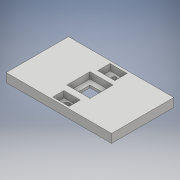
# Autodesk Inventor part: Parte8
Saved by Autodesk Inventor 2017 (Build 210142000, 142)
## iProperties
Part Number: Parte8
Material: Generico
Document SubType Name: Modeling
Designer: Federico
Density: 1 g/cm^3
Appearance: Default
Author: Federico
Autodesk Inventor part; units mm, degrees
ref_plane "YZ Plane" through (0, 0, 0) normal (1, 0, 0) x (0, 1, 0)
ref_plane "XZ Plane" through (0, 0, 0) normal (0, 1, 0) x (-1, 0, 0)
ref_plane "XY Plane" through (0, 0, 0) normal (0, 0, 1) x (1, 0, 0)
sketch "Schizzo1" plane through (0, 0, 0) normal (0, 0, 1) x (1, 0, 0)
  line L0 (-55, 32.5) -> (55, 32.5)
  line L1 (55, 32.5) -> (55, -32.5)
  line L2 (55, -32.5) -> (-55, -32.5)
  line L3 (-55, -32.5) -> (-55, 32.5)
  line L4 (-55, 32.5) -> (55, -32.5) construction
  line L5 (55, 32.5) -> (-55, -32.5) construction
  line L6 (-8.5, -18.7) -> (8.5, -18.7)
  line L7 (8.5, -18.7) -> (8.5, -30.3)
  line L8 (8.5, -30.3) -> (-8.5, -30.3)
  line L9 (-8.5, -30.3) -> (-8.5, -18.7)
  line L10 (-8.5, -18.7) -> (8.5, -30.3) construction
  line L11 (8.5, -18.7) -> (-8.5, -30.3) construction
  line L12 (-12, 12) -> (12, 12)
  line L13 (12, 12) -> (12, -12)
  line L14 (12, -12) -> (-12, -12)
  line L15 (-12, -12) -> (-12, 12)
  line L16 (-12, 12) -> (12, -12) construction
  line L17 (12, 12) -> (-12, -12) construction
  line L18 (-8.95, 29.85) -> (8.95, 29.85)
  line L19 (8.95, 29.85) -> (8.95, 17)
  line L20 (8.95, 17) -> (-8.95, 17)
  line L21 (-8.95, 17) -> (-8.95, 29.85)
  line L22 (-8.95, 29.85) -> (8.95, 17) construction
  line L23 (8.95, 29.85) -> (-8.95, 17) construction
  line L24 (0, 25.425) -> (0, 21.425) construction
  line L25 (-2, 25.425) -> (-2, 21.425)
  line L26 (2, 21.425) -> (2, 25.425)
  arc A0 (2, 25.425) -> (-2, 25.425) centre (0, 25.425) ccw
  arc A1 (-2, 21.425) -> (2, 21.425) centre (0, 21.425) ccw
  circle A2 centre (0, -24.5) radius 4.1
  circle A3 centre (0, 0) radius 3.8
  line L27 (-4, 4) -> (4, 4)
  line L28 (4, 4) -> (4, -4)
  line L29 (4, -4) -> (-4, -4)
  line L30 (-4, -4) -> (-4, 4)
  line L31 (-4, 4) -> (4, -4) construction
  line L32 (4, 4) -> (-4, -4) construction
  point P0 (0, 23.425)
  dimension "d0" = 110
  dimension "d1" = 65
  dimension "d5" = 17
  dimension "d6" = 11.6
  dimension "d8" = 24
  dimension "d9" = 24
  dimension "d11" = 17.9
  dimension "d12" = 12.85
  dimension "d13" = 2
  dimension "d14" = 4
  dimension "d15" = 8.2
  dimension "d16" = 7.6
  dimension "d17" = 8
  dimension "d18" = 8
  constraints: 68 end point, 11 parallel, 10 midpoint, 5 horizontal, 5 perpendicular, 4 centre point, 4 point on circle, 4 tangent, 1 coincident, 1 vertical
  measures "d0" distance of L1.end L2.end
  measures "d1" distance of L0.end L1.end
  measures "d5" distance of L7.end L8.end
  measures "d6" distance of L6.end L7.end
  measures "d8" distance of L13.end L14.end
  measures "d9" distance of L12.end L13.end
  measures "d11" distance of L19.end L20.end
  measures "d12" distance of L18.end L19.end
  measures "d13" distance of point (0, 23.425) L24.end
  measures "d14" diameter of A1
  measures "d15" diameter of A2
  measures "d16" diameter of A3
  measures "d17" distance of L28.end L29.end
  measures "d18" distance of L27.end L28.end
extrude "Estrusione1" add sketch "Schizzo1" along normal blind 9 contours L0 L1 L2 L3
sketch "Schizzo2" plane through (0, 0, 0) normal (0, 0, -1) x (-1, 0, 0)
  line L0 (-55, 32.5) -> (55, 32.5)
  line L1 (55, 32.5) -> (55, -32.5)
  line L2 (55, -32.5) -> (-55, -32.5)
  line L3 (-55, -32.5) -> (-55, 32.5)
  line L4 (-8.5, -18.7) -> (8.5, -18.7)
  line L5 (8.5, -18.7) -> (8.5, -30.3)
  line L6 (8.5, -30.3) -> (-8.5, -30.3)
  line L7 (-8.5, -30.3) -> (-8.5, -18.7)
  line L8 (-8.5, -18.7) -> (8.5, -30.3) construction
  line L9 (8.5, -18.7) -> (-8.5, -30.3) construction
  line L10 (-12, 12) -> (12, 12)
  line L11 (12, 12) -> (12, -12)
  line L12 (12, -12) -> (-12, -12)
  line L13 (-12, -12) -> (-12, 12)
  line L14 (-8.95, 29.85) -> (8.95, 29.85)
  line L15 (8.95, 29.85) -> (8.95, 17)
  line L16 (8.95, 17) -> (-8.95, 17)
  line L17 (-8.95, 17) -> (-8.95, 29.85)
  line L18 (-8.95, 29.85) -> (8.95, 17) construction
  line L19 (8.95, 29.85) -> (-8.95, 17) construction
  line L20 (0, 25.425) -> (0, 21.425) construction
  line L21 (-2, 25.425) -> (-2, 21.425)
  line L22 (2, 21.425) -> (2, 25.425)
  arc A0 (2, 25.425) -> (-2, 25.425) centre (0, 25.425) ccw
  arc A1 (-2, 21.425) -> (2, 21.425) centre (0, 21.425) ccw
  circle A2 centre (0, -24.5) radius 4.1
  line L23 (6.5, -6.5) -> (-6.5, -6.5)
  line L24 (-6.5, -6.5) -> (-6.5, 6.5)
  line L25 (-6.5, 6.5) -> (6.5, 6.5)
  line L26 (6.5, 6.5) -> (6.5, -6.5)
  point P0 (0, 0)
  point P1 (0, 0)
  point P2 (0, 23.425)
  dimension "d21" = 110
  dimension "d22" = 65
  dimension "d23" = 17
  dimension "d24" = 11.6
  dimension "d25" = 24
  dimension "d26" = 24
  dimension "d27" = 17.9
  dimension "d28" = 12.85
  dimension "d29" = 2
  dimension "d30" = 4
  dimension "d31" = 8.2
  dimension "d37" = 13
  dimension "d38" = 13
  constraints: 56 end point, 11 parallel, 5 horizontal, 5 perpendicular, 4 midpoint, 4 point on circle, 4 tangent, 3 centre point, 1 vertical
  measures "d21" distance of L1.end L2.end
  measures "d22" distance of L0.end L1.end
  measures "d23" distance of L5.end L6.end
  measures "d24" distance of L4.end L5.end
  measures "d25" distance of L11.end L12.end
  measures "d26" distance of L10.end L11.end
  measures "d27" distance of L15.end L16.end
  measures "d28" distance of L14.end L15.end
  measures "d29" distance of point (0, 23.425) L20.end
  measures "d30" diameter of A1
  measures "d31" diameter of A2
  measures "d37" distance of L24.end L25.end
  measures "d38" distance of L23.end L24.end
extrude "Estrusione4" add sketch "Schizzo2" against normal blind 2.5 contours L4 L5 L6 L7 | L10 L11 L12 L13 | L14 L15 L16 L17
